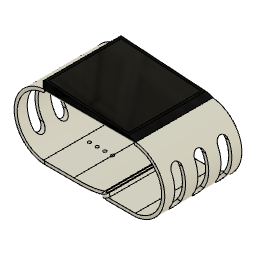
Smart watch SpaceApp Challenge v8 (Autodesk Fusion 360 design; units mm, degrees)
Autodesk Fusion 360 part; units mm, degrees
sketch "Sketch1" plane through (0, 0, 0) normal (0, 1, 0) x (1, 0, 0)
  arc A0 (-30, 30) -> (-30, -30) centre (-30, 0) ccw
  line L0 (-30, -30) -> (30, -30)
  arc A1 (30, -30) -> (30, 30) centre (30, 0) ccw
  line L1 (30, 0) -> (-30, 0) construction
  arc A2 (-30, 32) -> (-30, -32) centre (-30, 0) ccw
  line L2 (-30, -32) -> (30, -32)
  arc A3 (30, -32) -> (30, 32) centre (30, 0) ccw
  line L3 (30, 32) -> (30, 30)
  line L4 (-30, 32) -> (-30, 30)
  dimension "d1" = 2
  constraint tangent A0 L0
  constraint tangent L0 A1
  constraint horizontal L1
  constraint vertical L3
  constraint parallel L3 L4
extrude "Extrude1" add sketch "Sketch1" along normal mid plane 50 makes body 1 in component "Component"
sketch "Sketch2" plane through (0, 25, 0) normal (0, 1, 0) x (-1, 0, 0)
  line L0 (30, 32) -> (-30, 32)
  arc A0 (-30, 32) -> (-30, -32) centre (-30, 0) ccw
  line L1 (-30, -32) -> (-30, -30)
  arc A1 (-30, 30) -> (-30, -30) centre (-30, 0) ccw
  line L2 (-30, 30) -> (30, 30)
  arc A2 (30, -30) -> (30, 30) centre (30, 0) ccw
  arc A3 (30, -32) -> (30, 32) centre (30, 0) ccw
  line L3 (30, -30) -> (30, -32)
sketch "Sketch4" plane through (0, 25, 0) normal (0, 1, 0) x (-1, 0, 0)
  line L0 (30, 32) -> (-30, 32)
  arc A0 (-30, 32) -> (-30, -32) centre (-30, 0) ccw
  line L1 (-30, -32) -> (-30, -30)
  arc A1 (-30, 30) -> (-30, -30) centre (-30, 0) ccw
  line L2 (-30, 30) -> (30, 30)
  arc A2 (30, -30) -> (30, 30) centre (30, 0) ccw
  line L3 (30, -30) -> (30, -32)
  arc A3 (30, -32) -> (30, 32) centre (30, 0) ccw
  line L4 (30, 32) -> (30, 37)
  line L5 (30, 37) -> (-30, 33)
  line L6 (-30, 33) -> (-30, 32)
  dimension "d17" = 5
  dimension "d18" = 1
  constraint coincident L0.start A3.end
  constraint perpendicular L0 L4
  constraint coincident L0.end A0.start
  constraint perpendicular L0 L6
  measures "d17" distance of L0.start L4.end
  measures "d18" distance of L5.end L0.end
extrude "Extrude1'" add sketch "Sketch4" against normal blind 50 separate body contours L0 L4 L5 L6 makes body 2 in component "Component'"
fillet "Fillet1" radius 12 1 edges at (30, 0, 33) on bodies 2 in component "Component'"
fillet "Fillet2" radius 0.5 1 edges at (-30, 0, 37) on bodies 2 in component "Component'"
sketch "Sketch5" plane through (2.323, 0, 34.8451) normal (0.066519, 0, 0.997785) x (0, 1, 0)
  line L0 (25, 31.8603) -> (-25, 31.8603)
  line L1 (-25, 31.8603) -> (-25, -23.0142)
  line L2 (-25, -23.0142) -> (25, -23.0142)
  line L3 (25, -23.0142) -> (25, 31.8603)
  line L4 (23.5, -21.5142) -> (23.5, 30.3603)
  line L5 (23.5, 30.3603) -> (-23.5, 30.3603)
  line L6 (-23.5, 30.3603) -> (-23.5, -21.5142)
  line L7 (-23.5, -21.5142) -> (23.5, -21.5142)
  dimension "d23" = -1.5
extrude "Extrude2" cut sketch "Sketch5" against normal blind 0.5 contours L4 L5 L6 L7 bodies 2 in component "Component'"
sketch "Sketch6" plane through (-30, 0, 0) normal (-1, 0, 0) x (0, -1, 0)
  line L0 (25, 36.4656) -> (-25, 36.4656)
  line L1 (-25, 36.4656) -> (-25, 32)
  line L2 (-25, 32) -> (25, 32)
  line L3 (25, 32) -> (25, 36.4656)
  line L4 (-25, 36.4656) -> (25, 32) construction
  line L5 (25, 36.4656) -> (-25, 32) construction
  line L6 (5, 36) -> (-5, 36)
  line L7 (-5, 36) -> (-5, 32.4656)
  line L8 (-5, 32.4656) -> (5, 32.4656)
  line L9 (5, 32.4656) -> (5, 36)
  line L10 (5, 36) -> (-5, 32.4656) construction
  line L11 (-5, 36) -> (5, 32.4656) construction
  point P0 (0, 34.2328)
  constraint coincident L0.end L1.start
  constraint coincident L2.end L3.start
  constraint coincident L0.start L3.end
  constraint coincident L1.end L2.start
  constraint horizontal L6
  constraint perpendicular L6 L7
  constraint parallel L6 L8
  constraint parallel L7 L9
  constraint coincident L10 P0
  constraint coincident L11 P0
  constraint midpoint L4 P0
extrude "Extrude3" cut sketch "Sketch6" against normal blind 1 contours L6 L7 L8 L9 bodies 2 in component "Component'"
sketch "Sketch7" plane through (-29, 0, 0) normal (-1, 0, 0) x (0, -1, 0)
  line L0 (5, 32.4656) -> (5, 36)
  line L1 (5, 36) -> (-5, 36)
  line L2 (-5, 36) -> (-5, 32.4656)
  line L3 (-5, 32.4656) -> (5, 32.4656)
  line L4 (-5, 36) -> (5, 32.4656) construction
  line L5 (5, 36) -> (-5, 32.4656) construction
  circle A0 centre (0, 34.2328) radius 0.7672
  constraint coincident L1.end L2.start
  constraint coincident L0.start L3.end
  constraint coincident L0.end L1.start
  constraint coincident L2.end L3.start
  constraint midpoint L5 A0.centre
extrude "Extrude4" add sketch "Sketch7" along normal blind 0.7 contours A0 bodies 2 in component "Component'"
fillet "Fillet3" radius 0.75 1 edges at (-29.7, 0.7153, 33.9553) on bodies 2 in component "Component'"
sketch "Sketch8" plane through (0, 0, 30) normal (0, 0, -1) x (1, 0, 0)
  line L0 (-30, 25) -> (-30, -25)
  line L1 (-30, -25) -> (30, -25)
  line L2 (30, -25) -> (30, 25)
  line L3 (30, 25) -> (-30, 25)
  line L4 (-4.4231, 10.6154) -> (-10.4231, 14.6154)
  arc A0 (-10.4231, 14.6154) -> (-12.5769, 11.3846) centre (-11.5, 13) ccw
  line L5 (-12.5769, 11.3846) -> (-6.5769, 7.3846)
  arc A1 (-6.5769, 7.3846) -> (-4.4231, 10.6154) centre (-5.5, 9) ccw
  line L6 (-5.5, 9) -> (-11.5, 13) construction
  line L7 (0, 0) -> (-13.5, 0) construction
  line L8 (-12.5769, -11.3846) -> (-6.5769, -7.3846)
  arc A2 (-12.5769, -11.3846) -> (-10.4231, -14.6154) centre (-11.5, -13) ccw
  line L9 (-4.4231, -10.6154) -> (-10.4231, -14.6154)
  arc A3 (-4.4231, -10.6154) -> (-6.5769, -7.3846) centre (-5.5, -9) ccw
  circle A4 centre (-22, 4) radius 1
  circle A5 centre (-22, 0) radius 1
  circle A6 centre (-22, -4) radius 1
  line L10 (0, 0) -> (0, 4.5) construction
  line L11 (4.4231, 10.6154) -> (10.4231, 14.6154)
  line L12 (12.5769, 11.3846) -> (6.5769, 7.3846)
  arc A7 (4.4231, 10.6154) -> (6.5769, 7.3846) centre (5.5, 9) ccw
  arc A8 (12.5769, 11.3846) -> (10.4231, 14.6154) centre (11.5, 13) ccw
  arc A9 (6.5769, -7.3846) -> (4.4231, -10.6154) centre (5.5, -9) ccw
  line L13 (4.4231, -10.6154) -> (10.4231, -14.6154)
  line L14 (12.5769, -11.3846) -> (6.5769, -7.3846)
  arc A10 (10.4231, -14.6154) -> (12.5769, -11.3846) centre (11.5, -13) ccw
  point P0 (-8.5, 11)
  point P1 (0, 11)
  point P2 (-8.5, 11)
  constraint tangent L4 A0
  constraint tangent A0 L5
  constraint parallel L4 L5
  constraint tangent L5 A1
  constraint tangent L4 A1
  constraint midpoint L6 P2
  constraint coincident L7.start L10.start
  constraint horizontal L7
  constraint symmetric L4.start L7 L9.start
  constraint symmetric L4.end L7 A2.end
  constraint symmetric A0.end L7 L8.start
  constraint symmetric L5.end L7 L8.end
  constraint symmetric A0 L7 A2
  constraint symmetric A1 L7 A3
  constraint coincident P2 P0
  constraint perpendicular L7 L10
  constraint symmetric L4.start L10 L11.start
  constraint symmetric L4.end L10 L11.end
  constraint symmetric A0.end L10 L12.start
  constraint symmetric L5.end L10 L12.end
  constraint symmetric A0 L10 A8
  constraint symmetric A1 L10 A7
  constraint symmetric L8.start L10 L14.start
  constraint symmetric L8.end L10 A9.start
  constraint symmetric A2.end L10 L13.end
  constraint symmetric A2 L10 A10
  constraint symmetric L9.start L10 A9.end
  constraint symmetric A3 L10 A9
extrude "Extrude5" cut sketch "Sketch8" against normal blind 1.5 contours L4 A0 L5 A1 | L8 A2 L9 A3 | L11 L12 A7 A8 | A9 L13 L14 A10 bodies 1 in component "Component"
extrude "Extrude6" cut sketch "Sketch8" against normal blind 0.7 contours A4 | A5 | A6 bodies 1 in component "Component"
fillet "Fillet1'" radius 1 3 edges at (-22.9323, 3.6384, 30.7) (-22.9323, -0.3616, 30.7) (-22.9323, -4.3616, 30.7) on bodies 1 in component "Component"
split "Split1" by plane through (-30, 25, 32) normal (-1, 0, 0) bodies 1 makes body 3 at (-56.8808, -8.3333, 17.3615) in component "Component"
sketch "Sketch9" plane through (0, 25, 0) normal (0, 1, 0) x (-1, 0, 0)
  line L0 (30, 30) -> (30, 32)
  line L1 (30, 32) -> (-30, 32)
  arc A0 (-30, 32) -> (-30, -32) centre (-30, 0) ccw
  line L2 (-30, -32) -> (-30, -30)
  arc A1 (-30, 30) -> (-30, -30) centre (-30, 0) ccw
  line L3 (-30, 30) -> (30, 30)
  line L4 (30, 32) -> (67.4543, 32)
  line L5 (67.4543, 32) -> (67.4543, -32.8714)
  line L6 (67.4543, -32.8714) -> (30, -32.8714)
  line L7 (30, -32.8714) -> (30, 32)
  line L8 (-30, 32) -> (-65.0107, 32)
  line L9 (-65.0107, 32) -> (-65.0107, -32.8714)
  line L10 (-65.0107, -32.8714) -> (-30, -32.8714)
  line L11 (-30, -32.8714) -> (-30, 32)
  constraint horizontal L4
  constraint vertical L5
  constraint horizontal L6
  constraint vertical L7
  constraint coincident L0.end L1.start
  constraint horizontal L8
  constraint vertical L9
  constraint horizontal L10
  constraint vertical L11
  constraint coincident L1.end A0.start
extrude "Extrude7" cut sketch "Sketch9" against normal blind 55 contours L0 L4 L5 L6 L7 | A0 L2 A1 L11 bodies 1 3 in component "Component"
sketch "Sketch10" plane through (0, -25, 0) normal (0, -1, 0) x (1, 0, 0)
  line L0 (30, 30) -> (30, 32)
  line L1 (30, 32) -> (-30, 32)
  line L2 (-30, 32) -> (-30, 30)
  line L3 (-30, 30) -> (30, 30)
  circle A0 centre (-30, 31) radius 1
  circle A1 centre (30, 31) radius 1
  constraint midpoint L2 A0.centre
  constraint coincident L1.end A0
  constraint midpoint L0 A1.centre
  constraint coincident L0.end A1
extrude "Extrude8" cut sketch "Sketch10" against normal blind 50 contours L0 A1 | L2 A0 picked at (29.5429, 31.2078) picked at (-29.6968, 31.1385) bodies 1 in component "Component"
sketch "Sketch11" plane through (0, -25, 0) normal (0, -1, 0) x (1, 0, 0)
  arc A0 (-30, 30) -> (-30, 32) centre (-30, 31) ccw
  line L0 (-30, 30) -> (30, 30)
  arc A1 (30, 32) -> (30, 30) centre (30, 31) ccw
  line L1 (30, 32) -> (-30, 32)
  arc A2 (30, -10) -> (30, 32) centre (27.6571, 11) ccw
  arc A3 (29.7782, -8.0123) -> (29.7782, 30.0123) centre (27.6571, 11) ccw
  arc A4 (29.7782, -8.0123) -> (30, -10) centre (29.8891, -9.0062) ccw
  arc A5 (-30, 32) -> (-30, -10) centre (-27.6571, 11) ccw
  arc A6 (-29.7782, 30.0123) -> (-29.7782, -8.0123) centre (-27.6571, 11) ccw
  arc A7 (-30, 30) -> (-30, 32) centre (-30, 31) ccw
  arc A8 (-30, -10) -> (-29.7782, -8.0123) centre (-29.8891, -9.0062) ccw
  dimension "d41" = -2
  constraint coincident A1.start L1.start
  constraint tangent A3 A4
extrude "Extrude1''" add sketch "Sketch11" against normal blind 50 separate body contours A0 L0 A5 A6 A7 A8 makes body 4 in component "Component''"
extrude "Extrude1'''" add sketch "Sketch11" against normal blind 50 separate body contours L0 A1 A2 A3 A4 makes body 5 in component "Component'''"
sketch "Sketch12" plane through (0, 25, 0) normal (0, 1, 0) x (-1, 0, 0)
  arc A0 (30, 32) -> (30, 30) centre (30, 31) ccw
  line L0 (30, 30) -> (29.886, 30)
  arc A1 (29.7782, -8.0123) -> (29.886, 30) centre (27.6571, 11) ccw
  arc A2 (29.7782, -8.0123) -> (30, -10) centre (29.8891, -9.0062) ccw
  arc A3 (30, -10) -> (30, 32) centre (27.6571, 11) ccw
  line L1 (29.7782, -8.0123) -> (10.0874, -8.0123)
  line L2 (10.0874, -8.0123) -> (10.0874, -10.0123)
  line L3 (10.0874, -10.0123) -> (29.7782, -10.0123)
  line L4 (29.7782, -10.0123) -> (29.7782, -8.0123)
  spline S0 degree 5 poles (10.0874, -8.0123) (9.5103, -8.0123) (8.3702, -8.0072) (6.702, -7.9839) (4.5633, -7.9213) (2.0421, -7.7868) (-0.3132, -7.5911) (-2.4892, -7.3291) (-4.4781, -6.9978) (-6.2879, -6.6002) (-7.9483, -6.1469) (-9.1841, -5.7497) (-10.072, -5.437) (-10.6482, -5.2226) (-10.9324, -5.1139) knots 0 0 0 0 0 0 0.1 0.2 0.3 0.4 0.5 0.6 0.7 0.8 0.9 1 1 1 1 1 1
  spline S1 degree 3 poles (10.0874, -10.0123) (5.184, -10.0123) (0.8316, -9.8042) (-2.8016, -9.2808) (-5.9591, -8.8259) (-8.5152, -8.1142) (-10.7573, -7.3112) (-11.0586, -7.2033) (-11.3549, -7.0936) (-11.6469, -6.9819) knots 0 0 0 0 0.503551 0.503551 0.503551 0.941187 0.941187 0.941187 1 1 1 1
  arc A4 (-10.9324, -5.1139) -> (-11.6469, -6.9819) centre (-11.2897, -6.0479) ccw
  line L5 (-9.1105, -5.8107) -> (-12.7544, -4.417)
  point P0 (-3.9217, -7.0758)
  dimension "d49" = -2
  constraint horizontal L1
  constraint vertical L2
  constraint horizontal L3
  constraint vertical L4
  constraint coincident A1.start A2.start
  constraint tangent S0 A4
  constraint coincident L2.end L3.start
  constraint midpoint S0.end L5
extrude "Extrude9" add sketch "Sketch12" against normal blind 50 contours A2 L1 L2 L3 L4 | L2 S0 S1 A4 bodies 3 in component "Component"
ref_plane "WorkPlane3" through (10.9324, 0, -5.1139) normal (-0.34202, 0, 0.939693) x (0, -1, 0)
sketch "Sketch13" plane through (10.9324, 0, -5.1139) normal (-0.34202, 0, 0.939693) x (0, -1, 0)
  line L0 (26, 3) -> (-26, 3)
  line L1 (-26, 3) -> (-26, -1)
  line L2 (-26, -1) -> (26, -1)
  line L3 (26, -1) -> (26, 3)
  arc A0 (-26, 3) -> (-26, -1) centre (-26, 1) ccw
  arc A1 (26, -1) -> (26, 3) centre (26, 1) ccw
  dimension "d55" = 4
  constraint horizontal L0
  constraint vertical L1
  constraint horizontal L2
  constraint vertical L3
  constraint tangent L0 A0
  constraint tangent L0 A1
  measures "d55" distance of L0 L2
extrude "Extrude10" add sketch "Sketch13" against normal blind 2 bodies 3 in component "Component"
sketch "Sketch14" plane through (2.9224, 0, -8.0293) normal (-0.34202, 0, 0.939693) x (0, -1, 0)
  arc A0 (26, 7.5241) -> (26, 11.5241) centre (26, 9.5241) ccw
  line L0 (26, 11.5241) -> (-26, 11.5241)
  arc A1 (-26, 11.5241) -> (-26, 7.5241) centre (-26, 9.5241) ccw
  line L1 (-26, 7.5241) -> (26, 7.5241)
  line L2 (-25, 8.5565) -> (25, 8.5565)
  line L3 (25, 8.5565) -> (25, 8.5241)
  line L4 (25, 8.5241) -> (-25, 8.5241)
  line L5 (-25, 8.5241) -> (-25, 8.5565)
  line L6 (25, 8.5565) -> (-24.9198, 8.5565)
  line L7 (-24.9198, 8.5565) -> (-24.9198, 10.5565)
  line L8 (-24.9198, 10.5565) -> (25, 10.5565)
  line L9 (25, 10.5565) -> (25, 8.5565)
  arc A2 (-24.9198, 10.5565) -> (-25, 8.5565) centre (-24.9198, 9.5549) ccw
  arc A3 (25, 8.5565) -> (25, 10.5565) centre (25, 9.5565) ccw
  dimension "d56" = 2
  constraint horizontal L6
  constraint vertical L7
  constraint horizontal L8
  constraint vertical L9
  constraint coincident L2.end L3.start
  constraint coincident L2.start L5.end
  constraint tangent L8 A2
  constraint tangent L8 A3
  measures "d56" distance of L2.end L8.end
extrude "Extrude11" cut sketch "Sketch14" against normal blind 2 contours L2 L7 A2 | L2 L6 L7 L8 L9 | L9 A3 bodies 3 in component "Component"
sketch "Sketch15" plane through (0, -25, 0) normal (0, -1, 0) x (1, 0, 0)
  arc A0 (29.7782, -8.0123) -> (29.886, 30) centre (27.6571, 11) ccw
  arc A1 (29.7782, -8.0123) -> (30, -10) centre (29.8891, -9.0062) ccw
  arc A2 (30, -10) -> (30, 32) centre (27.6571, 11) ccw
  arc A3 (30, 32) -> (30, 30) centre (30, 31) ccw
  line L0 (30, 30) -> (29.886, 30)
  line L1 (29.7782, -8.0123) -> (11, -8.0123)
  line L2 (11, -8.0123) -> (11, -10)
  line L3 (11, -10) -> (29.7782, -10)
  line L4 (29.7782, -10) -> (29.7782, -8.0123)
  arc A4 (11, -8.0123) -> (11, -10) centre (11, -9.0062) ccw
  constraint horizontal L1
  constraint vertical L2
  constraint horizontal L3
  constraint vertical L4
  constraint coincident A0.start A1.start
  constraint tangent L1 A4
extrude "Extrude2'" add sketch "Sketch15" against normal blind 50 contours A1 L1 L2 L3 | L2 A4 bodies 5 in component "Component'''"
sketch "Sketch16" plane through (0, 0, 0) normal (1, 0, 0) x (0, 1, 0)
  line L0 (18.5, 0) -> (18.5, 20)
  arc A0 (18.5, 20) -> (11.5, 20) centre (15, 20) ccw
  line L1 (11.5, 20) -> (11.5, 0)
  arc A1 (11.5, 0) -> (18.5, 0) centre (15, 0) ccw
  line L2 (15, 0) -> (15, 20) construction
  line L3 (0, 0) -> (0, 5) construction
  line L4 (-11.5, 20) -> (-11.5, 0)
  line L5 (-18.5, 0) -> (-18.5, 20)
  arc A2 (-11.5, 20) -> (-18.5, 20) centre (-15, 20) ccw
  arc A3 (-18.5, 0) -> (-11.5, 0) centre (-15, 0) ccw
  line L6 (-3.5, 0) -> (-3.5, 20)
  line L7 (3.5, 0) -> (3.5, 20)
  arc A4 (3.5, 20) -> (-3.5, 20) centre (0, 20) ccw
  arc A5 (-3.5, 0) -> (3.5, 0) centre (0, 0) ccw
  point P0 (15, 10)
  dimension "d61" = 7
  dimension "d62" = 10
  dimension "d63" = 3.5
  constraint tangent L0 A0
  constraint tangent A0 L1
  constraint parallel L0 L1
  constraint tangent L1 A1
  constraint tangent L0 A1
  constraint vertical L2
  constraint midpoint L2 P0
  constraint coincident L3.start A5.centre
  constraint vertical L3
  constraint symmetric L0.start L3 L5.start
  constraint symmetric L0.end L3 L5.end
  constraint symmetric A0.end L3 L4.start
  constraint symmetric L1.end L3 L4.end
  constraint symmetric A0 L3 A2
  constraint symmetric A1 L3 A3
  constraint vertical L6
  constraint tangent L7 A4
  constraint tangent L6 A4
  constraint tangent L7 A5
  measures "d61" diameter of A0
  measures "d62" distance of A0.centre P0
  measures "d63" distance of L4 A3.centre
extrude "Extrude2''" cut sketch "Sketch16" along normal mid plane 120 bodies 4 in component "Component''"
extrude "Extrude3'" cut sketch "Sketch16" along normal mid plane 120 bodies 5 in component "Component'''"
sketch "Sketch17" plane through (0, 0, -10.0123) normal (0, 0, -1) x (1, 0, 0)
  line L0 (-29.7782, -25) -> (-10.0874, -25)
  line L1 (-10.0874, -25) -> (-10.0874, 25)
  line L2 (-10.0874, 25) -> (-29.7782, 25)
  line L3 (-29.7782, 25) -> (-29.7782, -25)
  line L4 (0, 0) -> (0, 6) construction
  circle A0 centre (-25, 0) radius 1
  circle A1 centre (-20, 0) radius 1
  circle A2 centre (-15, 0) radius 1
  circle A3 centre (-10.0874, 0) radius 1
  circle A4 centre (15, 0) radius 1
  circle A5 centre (20, 0) radius 1
  circle A6 centre (25, 0) radius 1
  dimension "d70" = 2
  constraint coincident L4.start origin
  constraint vertical L4
  constraint midpoint L1 A3.centre
  measures "d70" diameter of A3
extrude "Extrude12" cut sketch "Sketch17" against normal blind 2 contours L1 A3 | L1 A3 | A0 | A1 | A2 bodies 3 in component "Component"
extrude "Extrude1''''" add sketch "Sketch17" along normal blind 2 separate body contours A4 | A5 | A6 makes body 6 at (25.3185, -0.9479, -11.3457) makes body 7 at (20.3185, -0.9479, -11.3457) makes body 8 at (15.995, 0.0996, -11.3457)
fillet "Fillet1''" radius 1 3 edges at (24.0677, 0.3616, -12.0123) (19.0677, 0.3616, -12.0123) (14.0677, 0.3616, -12.0123) on bodies 6 7 8
surface "SurfacePatch1" add patch along 4 edges at (-2.0903, -23.5, 35.1394) (-27.9701, 0, 36.8647) (-2.0903, 23.5, 35.1394) (23.7896, 0, 33.414) separate body on bodies 2 makes body 9
surface "SurfacePatch2" add patch along 4 edges at (9.5769, 9.3846, 30) (13.1154, 14.0769, 30) (7.4231, 12.6154, 30) (3.8846, 7.9231, 30) separate body on bodies 1 makes body 10
surface "SurfacePatch3" add patch along 4 edges at (7.4231, -12.6154, 30) (13.1154, -14.0769, 30) (9.5769, -9.3846, 30) (3.8846, -7.9231, 30) separate body on bodies 1 makes body 11
surface "SurfacePatch4" add patch along 4 edges at (-13.1154, 14.0769, 30) (-9.5769, 9.3846, 30) (-3.8846, 7.9231, 30) (-7.4231, 12.6154, 30) separate body on bodies 1 makes body 12
surface "SurfacePatch5" add patch along 4 edges at (-7.4231, -12.6154, 30) (-3.8846, -7.9231, 30) (-9.5769, -9.3846, 30) (-13.1154, -14.0769, 30) separate body on bodies 1 makes body 13
surface "SurfacePatch6" add patch along 4 edges at (-30, 5, 34.2328) (-30, 0, 36) (-30, -5, 34.2328) (-30, 0, 32.4656) separate body on bodies 2 makes body 14
fillet "Fillet2'" radius 2 2 edges at (0, -25, 30) (0, 25, 30) on bodies 1 in component "Component"
component "Component" placed x (1, 0, 0) y (0, 1, 0) z (0, 0, 1) at (0, 0, 0)
component "Component'" placed x (1, 0, 0) y (0, 1, 0) z (0, 0, 1) at (0, 0, 0)
component "Component''" placed x (1, 0, 0) y (0, 1, 0) z (0, 0, 1) at (0, 0, 0)
component "Component'''" placed x (1, 0, 0) y (0, 1, 0) z (0, 0, 1) at (0, 0, 0)
